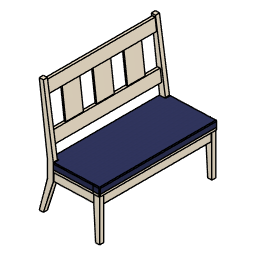
Slatback Bench 2020 (Autodesk Fusion 360 design; units mm, degrees)
Autodesk Fusion 360 part; units mm, degrees
note: some values were not read from the file. Chosen so that the rebuilt part matches the saved one: a direction. Set by a fixed rule: which sketch regions a step uses.
sketch "Sketch1" plane through (0, 0, 0) normal (0, 0, 1) x (1, 0, 0) in component "RearPost"
  line L0 (0, 0) -> (34.925, 0)
  line L1 (121.1545, 271.4692) -> (121.1545, 417.6082)
  line L2 (34.925, 990.6) -> (0, 990.6)
  line L3 (0, 990.6) -> (0, 0)
  line L4 (34.925, 990.6) -> (121.1545, 417.6082)
  line L5 (121.1545, 271.4692) -> (34.925, 0)
  line L6 (34.925, 990.6) -> (34.925, 0) construction
  line L7 (108.7337, 990.6) -> (34.925, 990.6) construction
  line L8 (34.925, 0) -> (111.2989, 0) construction
  line L9 (121.1545, 417.6082) -> (108.7337, 990.6) construction
  line L10 (111.2989, 0) -> (121.1545, 271.4692) construction
  line L11 (0, 990.6) -> (70.3545, 417.6082)
  line L12 (70.3545, 417.6082) -> (70.3545, 271.4692)
  line L13 (70.3545, 271.4692) -> (0, 0)
  line L14 (121.1545, 271.4692) -> (70.3545, 271.4692) construction
  line L15 (70.3545, 417.6082) -> (121.1545, 417.6082) construction
  dimension "d89" = 990.6
  dimension "d91" = 34.925
  dimension "d95" = 417.6082
  dimension "d97" = 50.8
  dimension "d189" = 121.1545
  dimension "d266" = 0
  dimension "d267" = 0
  dimension "d268" = 0
  dimension "d269" = 0
  dimension "d500" = 0
  dimension "d501" = 0
  dimension "d502" = 0
  dimension "d503" = 0
  dimension "d512" = 0
  dimension "d513" = 0
  dimension "d514" = 0
  dimension "d515" = 0
  dimension "d554" = 0
  dimension "d555" = 0
  dimension "d556" = 0
  dimension "d557" = 0
  dimension "d908" = 7
  constraint horizontal L0
  constraint horizontal L2
  constraint vertical L3
  constraint coincident L0.start L3.end
  constraint perpendicular L0 L6
  constraint horizontal L7
  constraint horizontal L8
  constraint perpendicular L2 L12
  constraint horizontal L15
  constraint horizontal L14
  measures "d89" distance of L0.start L2.end
  measures "d91" distance of L2.end L2.start
  measures "d95" distance of L0 L1.end
  measures "d97" distance of L1 L12
  measures "d189" distance of L1 L3
  measures "d908" angle of L3 L11
extrude "Extrude1" add sketch "Sketch1" along normal blind 34.925 contours L0 L1 L2 L4 L5 L11 L12 L13 makes body 1 in component "RearPost"
ref_plane "WorkPlane1" through (60.5773, 495.3, 17.4625) normal (0, 0, 1) x (1, 0, 0) in component "RearPost"
ref_plane "WorkPlane2" through (121.1545, 419.9193, 17.4625) normal (-0.000175, 0, 1) x (0, 1, 0) in component "RearPost"
sketch "Sketch1 (1)" plane through (121.1545, 419.9193, 17.4625) normal (-0.000175, 0, 1) x (0, 1, 0) in component "RearPost"
  line L0 (-606.7514, 0) -> (606.7514, 0)
  line L1 (-142.0963, 0) -> (-142.9054, 23.1684)
  line L2 (-142.9054, 23.1684) -> (-79.444, 25.3845)
  line L3 (-79.444, 25.3845) -> (-78.5576, 0)
  line L4 (-78.5576, 0) -> (-77.6711, -25.3845)
  line L5 (-77.6711, -25.3845) -> (-141.1325, -27.6006)
  line L6 (-141.1325, -27.6006) -> (-142.0963, 0)
  line L7 (-148.4502, 0.003) -> (-148.4502, -0.003)
  dimension "d221" = 92
  dimension "d224" = 63.5
  dimension "d237" = 25.4
  dimension "d574" = 25.4
  constraint coincident L0 L1.start
  constraint perpendicular L1 L2
  constraint coincident L0 L3.end
  constraint perpendicular L2 L3
  constraint perpendicular L4 L5
  constraint parallel L1 L6
  constraint parallel L3 L4
  measures "d221" angle of L0 L1
  measures "d224" distance of L1.end L2.end
  measures "d237" distance of L2.end L3.end
  measures "d574" distance of L3.end L4.end
extrude "Extrude2" cut sketch "Sketch1 (1)" along normal mid plane 12.7 bodies 1 in component "RearPost"
sketch "Sketch3" plane through (0, 0, 0) normal (0, 0, -1) x (-1, 0, 0) in component "RearPost"
  line L0 (0, 990.6) -> (-34.925, 990.6)
  line L1 (-34.925, 990.6) -> (-121.1545, 417.6082)
  line L2 (-121.1545, 417.6082) -> (-121.1545, 271.4692)
  line L3 (-121.1545, 271.4692) -> (-34.925, 0)
  line L4 (-34.925, 0) -> (0, 0)
  line L5 (0, 0) -> (-70.3545, 271.4692)
  line L6 (-70.3545, 271.4692) -> (-70.3545, 417.6082)
  line L7 (-70.3545, 417.6082) -> (0, 990.6)
  line L8 (-121.1545, 271.4692) -> (-70.3545, 271.4692) construction
  line L9 (-94.167, 341.3192) -> (-81.467, 341.3192)
  line L10 (-81.467, 341.3192) -> (-81.467, 277.8192)
  line L11 (-81.467, 277.8192) -> (-94.167, 277.8192)
  line L12 (-94.167, 277.8192) -> (-94.167, 341.3192)
  dimension "d110" = 11.1125
  dimension "d111" = 12.7
  dimension "d112" = 6.35
  dimension "d113" = 63.5
  constraint coincident L2.end L3.start
  constraint coincident L5.end L6.start
  constraint horizontal L9
  constraint vertical L10
  constraint horizontal L11
  constraint vertical L12
  measures "d110" distance of L6 L10
  measures "d111" distance of L9.start L9.end
  measures "d112" distance of L8 L11
  measures "d113" distance of L9.end L10.end
extrude "Extrude3" cut sketch "Sketch3" against normal blind 25.4 contours L9 L10 L11 L12 bodies 1 in component "RearPost"
sketch "Sketch2" plane through (0, 0, 0) normal (0, 0, -1) x (-1, 0, 0) in component "RearPost"
  line L0 (-81.467, 341.3192) -> (-81.467, 277.8192)
  line L1 (-81.467, 277.8192) -> (-94.167, 277.8192)
  line L2 (-94.167, 277.8192) -> (-94.167, 341.3192)
  line L3 (-94.167, 341.3192) -> (-81.467, 341.3192)
  line L4 (0, 990.6) -> (-34.925, 990.6)
  line L5 (-34.925, 990.6) -> (-121.1545, 417.6082)
  line L6 (-121.1545, 417.6082) -> (-121.1545, 271.4692)
  line L7 (-121.1545, 271.4692) -> (-34.925, 0)
  line L8 (-34.925, 0) -> (0, 0)
  line L9 (0, 0) -> (-70.3545, 271.4692)
  line L10 (-70.3545, 271.4692) -> (-70.3545, 417.6082)
  line L11 (-70.3545, 417.6082) -> (0, 990.6)
  line L12 (-81.6076, 521.3529) -> (-70.7734, 609.5902)
  line L13 (-70.7734, 609.5902) -> (-58.1681, 608.0425)
  line L14 (-58.1681, 608.0425) -> (-69.0023, 519.8052)
  line L15 (-69.0023, 519.8052) -> (-81.6076, 521.3529)
  line L16 (-121.1545, 417.6082) -> (-70.3545, 417.6082) construction
  line L17 (-69.0023, 519.8052) -> (-81.3842, 418.9625) construction
  line L18 (-37.5647, 880.054) -> (-26.7305, 968.2913)
  line L19 (-14.1252, 966.7436) -> (-24.9593, 878.5062)
  line L20 (-26.7305, 968.2913) -> (-14.1252, 966.7436)
  line L21 (-24.9593, 878.5062) -> (-37.5647, 880.054)
  line L22 (-58.1681, 608.0425) -> (-24.9593, 878.5062) construction
  line L23 (-14.1252, 966.7436) -> (-11.0297, 991.9543) construction
  line L24 (-70.3545, 417.6082) -> (-81.3842, 418.9625) construction
  line L25 (0, 990.6) -> (-11.0297, 991.9543) construction
  dimension "d852" = 12.7
  dimension "d853" = 88.9
  dimension "d854" = 101.6
  dimension "d857" = 11.1125
  dimension "d860" = 12.7
  dimension "d861" = 88.9
  dimension "d862" = 25.4
  constraint perpendicular L12 L13
  constraint perpendicular L13 L14
  constraint perpendicular L14 L15
  constraint parallel L11 L14
  constraint coincident L5.end L6.start
  constraint coincident L10.end L11.start
  constraint perpendicular L15 L17
  constraint perpendicular L18 L20
  constraint perpendicular L19 L20
  constraint perpendicular L19 L21
  constraint collinear L14 L22
  constraint collinear L19 L22
  constraint perpendicular L20 L23
  constraint perpendicular L11 L24
  constraint coincident L17.end L24.end
  constraint coincident L4.start L11.end
  constraint perpendicular L11 L25
  constraint coincident L23.end L25.end
  measures "d852" distance of L12 L14
  measures "d853" distance of L13.end L14.end
  measures "d854" distance of L14.end L17.end
  measures "d857" distance of L11 L14
  measures "d860" distance of L18 L19
  measures "d861" distance of L19.start L19.end
  measures "d862" distance of L19.start L23.end
extrude "Extrude3'" cut sketch "Sketch2" against normal blind 25.4 contours L12 L13 L14 L15 | L18 L19 L20 L21 bodies 1 in component "RearPost"
sketch "Sketch1 (2)" plane through (0, 0, 0) normal (0, 0, 1) x (1, 0, 0) in component "SideRail"
  line L0 (0, 0) -> (349.4629, 0)
  line L1 (349.4629, 0) -> (352.1238, 76.2)
  line L2 (352.1238, 76.2) -> (2.661, 76.2)
  line L3 (2.661, 76.2) -> (0, 0)
  dimension "d116" = 349.4629
  dimension "d169" = 88
  dimension "d209" = 76.2
  dimension "d262" = 0
  dimension "d263" = 0
  dimension "d264" = 0
  dimension "d265" = 0
  dimension "d496" = 0
  dimension "d497" = 0
  dimension "d498" = 0
  dimension "d499" = 0
  dimension "d508" = 0
  dimension "d509" = 0
  dimension "d510" = 0
  dimension "d511" = 0
  dimension "d550" = 0
  dimension "d551" = 0
  dimension "d552" = 0
  dimension "d553" = 0
  constraint horizontal L0
  constraint horizontal L2
  constraint coincident L0.start L3.end
  constraint parallel L1 L3
  measures "d116" distance of L0.start L0.end
  measures "d169" angle of L0 L3
  measures "d209" distance of L0 L2
sketch "Sketch4" plane through (0, 0, 0) normal (0, 1, 0) x (1, 0, 0) in component "SideRail"
  line L0 (0, 0) -> (-0.0044, 25.4)
  line L1 (352.1238, 0) -> (2.661, 0)
  line L2 (0, 0) -> (0, 25.4) construction
  line L3 (0, 25.4) -> (-0.0044, 25.4) construction
  dimension "d210" = 90.01
  dimension "d217" = 25.4
  constraint coincident L0.start L2.start
  constraint vertical L2
  constraint horizontal L3
  measures "d210" angle of L0 L1
  measures "d217" distance of L0.start L2.end
sweep "Sweep1" add profiles "Sketch1 (2)" path "Sketch4" along L0 section 1 separate body makes body 2 in component "SideRail"
ref_plane "WorkPlane2" through (176.0575, 38.1, -12.7) normal (0, 0, -1) x (-1, 0, 0) in component "SideRail"
sketch "Sketch3 (2)" plane through (179.1297, 38.0768, -12.7) normal (0, 0, -1) x (1, 0, 0) in component "SideRail"
  line L0 (-178.9101, 31.7268) -> (-202.0927, 31.7268)
  line L1 (-202.0927, 31.7268) -> (-202.0927, -31.7732)
  line L2 (-202.0927, -31.7732) -> (-176.6927, -31.7732)
  line L3 (170.5527, 31.7268) -> (195.9527, 31.7268)
  line L4 (195.9527, 31.7268) -> (195.9527, -31.7732)
  line L5 (195.9527, -31.7732) -> (172.7702, -31.7732)
  line L6 (172.9942, -38.1232) -> (172.9897, -38.1232)
  line L7 (170.3332, 38.0768) -> (170.3288, 38.0768)
  line L8 (172.992, -38.1232) -> (170.331, 38.0768)
  line L9 (-176.4687, -38.1232) -> (-176.4731, -38.1232)
  line L10 (-179.1297, 38.0768) -> (-179.1341, 38.0768)
  line L11 (-176.4709, -38.1232) -> (-179.1319, 38.0768)
  line L12 (-176.6927, -31.7732) -> (172.7702, -31.7732)
  line L13 (170.5527, 31.7268) -> (-178.9101, 31.7268)
  line L14 (195.9527, -31.7732) -> (195.9527, -38.1232)
  line L15 (195.9527, -38.1232) -> (160.4613, -38.1232)
  line L16 (160.4613, -38.1232) -> (160.4613, -31.7732)
  dimension "d274" = 25.4
  dimension "d325" = 6.35
  dimension "d326" = 6.35
  constraint perpendicular L0 L1
  constraint perpendicular L1 L2
  constraint perpendicular L3 L4
  constraint perpendicular L4 L5
  constraint collinear L0 L3
  constraint collinear L2 L5
  constraint equal L0 L5
  constraint horizontal L2
  constraint midpoint L6 L8.start
  constraint midpoint L7 L8.end
  constraint coincident L3.start L8
  constraint coincident L5.end L8
  constraint midpoint L9 L11.start
  constraint midpoint L10 L11.end
  constraint coincident L2.end L11
  constraint coincident L0.start L11
  constraint perpendicular L5 L14
  constraint perpendicular L14 L15
  constraint coincident L12 L16.end
  constraint perpendicular L12 L16
  constraint coincident L8.start L15
  measures "d274" distance of L1.end L2.end
  measures "d325" distance of L0 L11.end
  measures "d326" distance of L2 L11.start
extrude "Extrude3''" add sketch "Sketch3 (2)" along normal mid plane 12.7 bodies 2 in component "SideRail"
sketch "Sketch4 (2)" plane through (0, 0, 0) normal (0, 0, 1) x (1, 0, 0) in component "FrontPost"
  line L0 (0, 0) -> (34.925, 0)
  line L1 (50.8, 0) -> (50.8, 283.9296) construction
  line L2 (50.8, 360.176) -> (0, 361.95)
  line L3 (0, 361.95) -> (0, 0)
  line L4 (50.8, 283.9296) -> (34.925, 0)
  line L5 (50.8, 283.9296) -> (50.8, 360.176)
  line L6 (34.925, 0) -> (50.8, 0) construction
  dimension "d137" = 361.95
  dimension "d139" = 34.925
  dimension "d140" = 76.2464
  dimension "d190" = 88
  dimension "d191" = 50.8
  dimension "d316" = 50.831
  constraint horizontal L0
  constraint vertical L1
  constraint vertical L3
  constraint coincident L0.start L3.end
  constraint vertical L5
  constraint horizontal L6
  measures "d137" distance of L0.start L2.end
  measures "d139" distance of L0.start L0.end
  measures "d140" distance of L2.start L1.end
  measures "d190" angle of L2 L3
  measures "d191" distance of L3 L5
  measures "d316" distance of L2.start L2.end
extrude "Extrude1'" add sketch "Sketch4 (2)" along normal blind 34.925 separate body makes body 3 in component "FrontPost"
ref_plane "WorkPlane1" through (25.4, 180.975, 17.4625) normal (0, 0, 1) x (1, 0, 0) in component "FrontPost"
ref_plane "WorkPlane2" through (50.8, 251.5139, 17.4625) normal (-0.000175, 0, 1) x (0, 1, 0) in component "FrontPost"
sketch "Sketch2 (2)" plane through (50.8, 251.5139, 17.4625) normal (-0.000175, 0, 1) x (0, 1, 0) in component "FrontPost"
  line L0 (94.9658, 0) -> (95.7838, 23.4252)
  line L1 (95.7838, 23.4252) -> (39.6773, 25.3845)
  line L2 (39.6773, 25.3845) -> (38.7908, 0)
  line L3 (-204.4066, 0) -> (204.4066, 0)
  line L4 (94.9658, 0) -> (94.7884, -5.08)
  line L5 (94.7884, -5.08) -> (38.6134, -5.08)
  line L6 (38.6134, -5.08) -> (38.7908, 0)
  line L7 (146.522, 21.6534) -> (145.5884, -5.08)
  line L8 (94.7884, -5.08) -> (145.5884, -5.08)
  line L9 (95.7838, 23.4252) -> (146.522, 21.6534)
  line L10 (32.4157, 0.003) -> (32.4157, -0.003)
  dimension "d192" = 25.4
  dimension "d279" = 92
  dimension "d647" = 50.8
  constraint parallel L0 L2
  constraint perpendicular L0 L1
  constraint coincident L2.end L3
  constraint coincident L0.start L3
  constraint parallel L2 L6
  constraint parallel L0 L4
  constraint parallel L5 L8
  constraint horizontal L5
  constraint parallel L1 L9
  constraint parallel L0 L7
  measures "d192" distance of L1.end L2.end
  measures "d279" angle of L0 L3
  measures "d647" distance of L4.end L7.end
extrude "Extrude3'''" cut sketch "Sketch2 (2)" along normal mid plane 12.7 bodies 3 in component "FrontPost"
sketch "Sketch3 (3)" plane through (0, 0, 34.925) normal (0, 0, 1) x (1, 0, 0) in component "FrontPost"
  line L0 (50.8, 283.9296) -> (50.8, 360.176)
  line L1 (50.8, 360.176) -> (0, 361.95)
  line L2 (0, 361.95) -> (0, 0)
  line L3 (0, 0) -> (34.925, 0)
  line L4 (34.925, 0) -> (50.8, 283.9296)
  line L5 (0, 361.95) -> (54.2925, 361.95)
  line L6 (11.1125, 355.6) -> (23.8125, 355.6)
  line L7 (23.8125, 355.6) -> (23.8125, 292.1)
  line L8 (23.8125, 292.1) -> (11.1125, 292.1)
  line L9 (11.1125, 292.1) -> (11.1125, 355.6)
  line L10 (11.1125, 355.6) -> (11.1125, 361.95)
  line L11 (23.8125, 355.6) -> (23.8125, 361.95)
  dimension "d544" = 12.7
  dimension "d545" = 6.35
  dimension "d546" = 63.5
  dimension "d547" = 11.1125
  constraint coincident L1.end L2.start
  constraint perpendicular L2 L5
  constraint horizontal L6
  constraint vertical L7
  constraint horizontal L8
  constraint vertical L9
  constraint coincident L5 L10.end
  constraint perpendicular L5 L10
  constraint coincident L5 L11.end
  constraint perpendicular L5 L11
  measures "d544" distance of L6.start L6.end
  measures "d545" distance of L5 L6
  measures "d546" distance of L6.start L8.end
  measures "d547" distance of L2 L9
extrude "Extrude4" cut sketch "Sketch3 (3)" against normal blind 25.4 contours L1 L6 L10 L11 | L1 L5 L10 L11 | L6 L7 L8 L9 bodies 3 in component "FrontPost"
sketch "Sketch3 (4)" plane through (0, 0, 0) normal (0, 0, 1) x (1, 0, 0) in component "FrontRail"
  line L0 (0, 0) -> (0, 74.925)
  line L1 (0, 74.925) -> (25.4, 75.8119)
  line L2 (25.4, 75.8119) -> (25.4, 0)
  line L3 (25.4, 0) -> (0, 0)
  line L4 (36.5125, 0) -> (36.5125, 76.2) construction
  line L5 (36.5125, 76.2) -> (-4.1275, 76.2) construction
  dimension "d669" = 25.4
  dimension "d670" = 11.1125
  dimension "d671" = 88
  dimension "d672" = 76.2
  constraint coincident L0.start L3.end
  constraint vertical L0
  constraint parallel L0 L2
  constraint perpendicular L0 L3
  constraint vertical L4
  constraint perpendicular L4 L5
  constraint coincident L1 L4.end
  constraint coincident L3 L4.start
  measures "d669" distance of L2.end L0.start
  measures "d670" distance of L2 L4
  measures "d671" angle of L1 L2
  measures "d672" distance of L4.start L4.end
extrude "Extrude3''''" add sketch "Sketch3 (4)" along normal blind 933.45 separate body makes body 4 in component "FrontRail"
ref_plane "WorkPlane2" through (12.7, 37.906, 466.725) normal (0, 0, 1) x (1, 0, 0) in component "FrontRail"
sketch "Sketch4 (3)" plane through (0, 0, 933.45) normal (0, 0, 1) x (1, 0, 0) in component "FrontRail"
  line L0 (25.4, 0) -> (25.4, 75.8119)
  line L1 (25.4, 75.8119) -> (0, 74.925)
  line L2 (0, 74.925) -> (0, 0)
  line L3 (0, 0) -> (25.4, 0)
  line L4 (6.35, 75.1467) -> (6.35, 6.35)
  line L5 (6.35, 6.35) -> (19.05, 6.35)
  line L6 (19.05, 6.35) -> (19.05, 75.5902)
  line L7 (12.7, 75.3685) -> (12.7, 0) construction
  point P0 (12.7, 6.35)
  dimension "d675" = 12.7
  dimension "d676" = 6.35
  constraint coincident L1 L4.start
  constraint parallel L0 L4
  constraint perpendicular L4 L5
  constraint coincident L1 L6.end
  constraint perpendicular L5 L6
  constraint midpoint L1 L7.start
  constraint midpoint L3 L7.end
  constraint midpoint L5 P0
  constraint coincident L7 P0
  measures "d675" distance of L4.end L5.end
  measures "d676" distance of L3 L5
extrude "Extrude4'" add sketch "Sketch4 (3)" along normal blind 25.4 contours L1 L4 L5 L6 bodies 4 in component "FrontRail"
mirror "Mirror2" about plane through (12.7, 37.906, 466.725) normal (0, 0, 1) of "Extrude4'" in component "FrontRail"
sketch "Sketch1 (3)" plane through (0, 0, 0) normal (0, 0, 1) x (1, 0, 0) in component "RearRail"
  line L0 (0, 0) -> (0, 74.8605)
  line L1 (0, 74.8605) -> (25.4, 75.7475)
  line L2 (25.4, 75.7475) -> (25.4, 0)
  line L3 (25.4, 0) -> (0, 0)
  line L4 (-11.1125, 113.0857) -> (-11.1125, 0) construction
  line L5 (-11.1125, 0) -> (39.6875, 0) construction
  line L6 (-11.1125, 113.0857) -> (39.6875, 113.0857) construction
  line L7 (39.6875, 0) -> (39.6875, 76.2464) construction
  line L8 (39.6875, 76.2464) -> (39.6875, 113.0857) construction
  dimension "d752" = 25.4
  dimension "d753" = 88
  dimension "d755" = 11.1125
  dimension "d756" = 50.8
  dimension "d757" = 76.2464
  constraint coincident L0.start L3.end
  constraint vertical L0
  constraint parallel L0 L2
  constraint perpendicular L0 L3
  constraint parallel L0 L4
  constraint perpendicular L4 L5
  constraint perpendicular L4 L6
  constraint collinear L3 L5
  constraint perpendicular L6 L8
  constraint coincident L1 L7.end
  constraint collinear L7 L8
  measures "d752" distance of L2.end L0.start
  measures "d753" angle of L1 L2
  measures "d755" distance of L0 L4
  measures "d756" distance of L4.end L5.end
  measures "d757" distance of L5.end L7.end
extrude "Extrude1''" add sketch "Sketch1 (3)" along normal blind 933.328 separate body makes body 5 in component "RearRail"
ref_plane "WorkPlane1" through (12.7, 37.8738, 466.664) normal (0, 0, 1) x (1, 0, 0) in component "RearRail"
sketch "Sketch2 (3)" plane through (0, 0, 933.328) normal (0, 0, 1) x (1, 0, 0) in component "RearRail"
  line L0 (25.4, 0) -> (25.4, 75.7475)
  line L1 (25.4, 75.7475) -> (0, 74.8605)
  line L2 (0, 74.8605) -> (0, 0)
  line L3 (0, 0) -> (25.4, 0)
  line L4 (6.35, 6.35) -> (19.05, 6.35)
  line L5 (19.05, 6.35) -> (19.05, 69.85)
  line L6 (19.05, 69.85) -> (6.35, 69.85)
  line L7 (6.35, 69.85) -> (6.35, 6.35)
  line L8 (12.7, 0) -> (12.7, 75.304) construction
  point P0 (12.7, 6.35)
  dimension "d760" = 6.35
  dimension "d761" = 12.7
  dimension "d762" = 63.5
  constraint horizontal L4
  constraint vertical L5
  constraint horizontal L6
  constraint vertical L7
  constraint midpoint L3 L8.start
  constraint midpoint L1 L8.end
  constraint midpoint L4 P0
  constraint coincident L8 P0
  measures "d760" distance of L3 L4
  measures "d761" distance of L4.start L4.end
  measures "d762" distance of L4.end L5.end
extrude "Extrude2'" add sketch "Sketch2 (3)" along normal blind 25.4 contours L4 L5 L6 L7 bodies 5 in component "RearRail"
mirror "Mirror1" about plane through (12.7, 37.8738, 466.664) normal (0, 0, 1) of "Extrude2'" in component "RearRail"
sketch "Sketch1 (4)" plane through (0, 0, 0) normal (0, 1, 0) x (1, 0, 0) in component "Seat"
  line L0 (0, 0) -> (52.4194, 0)
  line L1 (52.4194, 0) -> (52.4194, -41.275)
  line L2 (52.4194, -41.275) -> (401.9172, -41.336)
  line L3 (401.9172, 974.664) -> (52.4194, 974.603)
  line L4 (52.4194, 974.603) -> (52.4194, 933.328)
  line L5 (52.4194, 933.328) -> (0, 933.328)
  line L6 (0, 933.328) -> (0, 0)
  line L7 (401.9172, -41.336) -> (459.0672, -41.336)
  line L8 (459.0672, -41.336) -> (459.0672, 974.664)
  line L9 (459.0672, 974.664) -> (401.9172, 974.664)
  line L10 (401.9172, -41.336) -> (401.9172, 974.664) construction
  dimension "d780" = 90.01
  dimension "d781" = 90.01
  dimension "d785" = 933.328
  dimension "d786" = 52.4194
  dimension "d787" = 57.15
  dimension "d789" = 406.6477
  dimension "d790" = 1016
  constraint coincident L0.start L6.end
  constraint horizontal L0
  constraint perpendicular L0 L1
  constraint perpendicular L0 L6
  constraint collinear L1 L4
  constraint perpendicular L5 L6
  constraint equal L1 L4
  constraint perpendicular L7 L8
  constraint perpendicular L8 L9
  constraint parallel L8 L10
  constraint parallel L6 L8
  measures "d780" angle of L1 L2
  measures "d781" angle of L3 L4
  measures "d785" distance of L5.end L0.start
  measures "d786" distance of L0.start L0.end
  measures "d787" horizontal distance of L2.end L7.end
  measures "d789" distance of L1 L8
  measures "d790" distance of L7.end L8.end
sketch "Sketch2 (4)" plane through (0, 0, 0) normal (0, 0, 1) x (1, 0, 0) in component "Seat"
  line L0 (0, 0) -> (0.6652, 19.05)
  line L1 (0, 0) -> (0.045, 1.2883)
  line L2 (0, 19.05) -> (0.6652, 19.05) construction
  line L3 (0, 19.05) -> (0, 0) construction
  dimension "d791" = 19.05
  dimension "d792" = 2
  constraint coincident L0.start L1.start
  constraint coincident L0 L1.end
  constraint vertical L3
  constraint perpendicular L2 L3
  measures "d791" distance of L2.start L0.start
  measures "d792" angle of L0 L3
sweep "Sweep1'" add profiles "Sketch1 (4)" path "Sketch2 (4)" along L0 section 1 separate body makes body 6 in component "Seat"
fillet "Fillet1" radius 6.35 6 edges at (459.3998, 9.525, 41.336) (52.7521, 9.525, 41.275) (459.3998, 9.525, -974.664) (52.7521, 9.525, -974.603) (0.3326, 9.525, -933.328) (0.3326, 9.525, 0) on bodies 6 in component "Seat"
sketch "Sketch1 (5)" plane through (0, 0, 0) normal (0, 1, 0) x (1, 0, 0) in component "Cushion"
  line L0 (0, 0) -> (52.4194, 0)
  line L1 (52.4194, 0) -> (52.4194, -41.275)
  line L2 (52.4194, -41.275) -> (401.9172, -41.336)
  line L3 (401.9172, 974.664) -> (52.4194, 974.603)
  line L4 (52.4194, 974.603) -> (52.4194, 933.328)
  line L5 (52.4194, 933.328) -> (0, 933.328)
  line L6 (0, 933.328) -> (0, 0)
  line L7 (401.9172, -41.336) -> (459.0672, -41.336)
  line L8 (459.0672, -41.336) -> (459.0672, 974.664)
  line L9 (459.0672, 974.664) -> (401.9172, 974.664)
  line L10 (401.9172, -41.336) -> (401.9172, 974.664) construction
  dimension "d780_1" = 90.01
  dimension "d781_1" = 90.01
  dimension "d785_1" = 933.328
  dimension "d786_1" = 52.4194
  dimension "d787_1" = 57.15
  dimension "d789_1" = 406.6477
  dimension "d790_1" = 1016
  constraint coincident L0.start L6.end
  constraint horizontal L0
  constraint perpendicular L0 L1
  constraint perpendicular L0 L6
  constraint collinear L1 L4
  constraint perpendicular L5 L6
  constraint equal L1 L4
  constraint perpendicular L7 L8
  constraint perpendicular L8 L9
  constraint parallel L8 L10
  constraint parallel L6 L8
  measures "d780_1" angle of L1 L2
  measures "d781_1" angle of L3 L4
  measures "d785_1" distance of L5.end L0.start
  measures "d786_1" distance of L0.start L0.end
  measures "d787_1" horizontal distance of L2.end L7.end
  measures "d789_1" distance of L1 L8
  measures "d790_1" distance of L7.end L8.end
sketch "Sketch2 (5)" plane through (0, 0, 0) normal (0, 0, 1) x (1, 0, 0) in component "Cushion"
  line L0 (0, 0) -> (1.774, 50.8)
  line L1 (0, 0) -> (0.045, 1.2883)
  line L2 (0, 50.8) -> (1.774, 50.8) construction
  line L3 (0, 50.8) -> (0, 0) construction
  dimension "d791_1" = 50.8
  dimension "d792_1" = 2
  constraint coincident L0.start L1.start
  constraint coincident L0 L1.end
  constraint vertical L3
  constraint perpendicular L2 L3
  measures "d791_1" distance of L2.start L0.start
  measures "d792_1" angle of L0 L3
sweep "Sweep1''" add profiles "Sketch1 (5)" path "Sketch2 (5)" along L0 section 1 separate body makes body 7 in component "Cushion"
fillet "Fillet1'" radius 6.35 16 edges at (228.9423, 50.8, 41.3055) (432.2661, 50.8, 41.336) (460.8411, 50.8, -466.664) (432.2661, 50.8, -974.664) (228.9423, 50.8, -974.6335) (54.1934, 50.8, -953.9655) (27.9837, 50.8, -933.328) (1.774, 50.8, -466.664) (27.9837, 50.8, 0) (54.1934, 50.8, 20.6375) (459.9541, 25.4, -974.664) (53.3064, 25.4, -974.603) (459.9541, 25.4, 41.336) (53.3064, 25.4, 41.275) (0.887, 25.4, 0) (0.887, 25.4, -933.328) on bodies 7 in component "Cushion"
sketch "Sketch1 (6)" plane through (0, 0, 0) normal (0, 1, 0) x (1, 0, 0) in component "BackRail"
  line L0 (0, 0) -> (25.4, 0)
  line L1 (25.4, 0) -> (25.4, -933.328)
  line L2 (25.4, -933.328) -> (0, -933.328)
  line L3 (0, -933.328) -> (0, 0)
  dimension "d940" = 933.328
  dimension "d941" = 25.4
  constraint horizontal L0
  constraint vertical L1
  constraint horizontal L2
  constraint vertical L3
  constraint coincident L0.start L3.end
  measures "d940" distance of L0.end L1.end
  measures "d941" distance of L0.start L0.end
extrude "Extrude1'''" add sketch "Sketch1 (6)" along normal blind 101.6 separate body makes body 8 in component "BackRail"
ref_plane "WorkPlane1" through (12.7, 50.8, 466.664) normal (0, 0, 1) x (1, 0, 0) in component "BackRail"
sketch "Sketch2 (6)" plane through (0, 0, 933.328) normal (0, 0, 1) x (1, 0, 0) in component "BackRail"
  line L0 (6.35, 95.25) -> (19.05, 95.25)
  line L1 (19.05, 95.25) -> (19.05, 6.35)
  line L2 (19.05, 6.35) -> (6.35, 6.35)
  line L3 (6.35, 6.35) -> (6.35, 95.25)
  line L4 (0, 0) -> (25.4, 101.6) construction
  line L5 (6.35, 95.25) -> (19.05, 6.35) construction
  line L6 (0, 101.6) -> (25.4, 101.6)
  point P0 (25.4, 101.6)
  dimension "d871" = 12.7
  dimension "d942" = 6.35
  constraint horizontal L0
  constraint vertical L1
  constraint horizontal L2
  constraint vertical L3
  constraint midpoint L4 L5
  constraint coincident L4.start origin
  constraint coincident P0 L4.end
  measures "d871" distance of L1.end L2.end
  measures "d942" distance of L0 L6
extrude "Extrude2''" add sketch "Sketch2 (6)" along normal blind 25.4 bodies 8 in component "BackRail"
mirror "Mirror1'" about plane through (12.7, 50.8, 466.664) normal (0, 0, 1) of "Extrude2''" in component "BackRail"
sketch "Sketch3 (5)" plane through (0, 101.6, 0) normal (0, 1, 0) x (-1, 0, 0) in component "BackRail"
  line L0 (0, 933.328) -> (-25.4, 933.328)
  line L1 (-25.4, 933.328) -> (-25.4, 0)
  line L2 (-25.4, 0) -> (0, 0)
  line L3 (0, 0) -> (0, 933.328)
  line L4 (-9.525, 539.689) -> (-15.875, 539.689)
  line L5 (-15.875, 539.689) -> (-15.875, 393.639)
  line L6 (-15.875, 393.639) -> (-9.525, 393.639)
  line L7 (-9.525, 393.639) -> (-9.525, 539.689)
  line L8 (-12.7, 933.328) -> (-12.7, 0) construction
  line L9 (-9.525, 539.689) -> (-15.875, 393.639) construction
  line L10 (-15.875, 660.339) -> (-9.525, 660.339)
  line L11 (-9.525, 806.389) -> (-15.875, 806.389)
  line L12 (-15.875, 806.389) -> (-15.875, 660.339)
  line L13 (-9.525, 806.389) -> (-15.875, 660.339) construction
  line L14 (-9.525, 660.339) -> (-9.525, 806.389)
  line L15 (-15.875, 126.939) -> (-9.525, 126.939)
  line L16 (-9.525, 272.989) -> (-15.875, 272.989)
  line L17 (-15.875, 272.989) -> (-15.875, 126.939)
  line L18 (-9.525, 272.989) -> (-15.875, 126.939) construction
  line L19 (-9.525, 126.939) -> (-9.525, 272.989)
  point P0 (-25412.7042, 466.725)
  point P1 (-25412.7042, 466.664)
  dimension "d943" = 6.35
  dimension "d944" = 146.05
  dimension "d947" = 266.7
  dimension "d948" = 0
  constraint horizontal L4
  constraint vertical L5
  constraint horizontal L6
  constraint vertical L7
  constraint midpoint L0 L8.start
  constraint midpoint L2 L8.end
  constraint midpoint L8 L9
  measures "d943" distance of L4.start L4.end
  measures "d944" distance of L4.start L6.end
extrude "Extrude3'''''" cut sketch "Sketch3 (5)" against normal blind 12.7 contours L4 L5 L6 L7 | L10 L11 L12 L14 | L15 L16 L17 L19 bodies 8 in component "BackRail"
sketch "Sketch1 (7)" plane through (0, 0, 0) normal (0, 1, 0) x (1, 0, 0) in component "BackPanel"
  line L0 (0.0114, 0) -> (12.7114, 0)
  line L1 (12.7114, 0) -> (12.7114, -152.4) construction
  line L2 (12.7114, -152.4) -> (0.0114, -152.4)
  line L3 (0, -152.4) -> (0, 0) construction
  arc A0 (12.7114, 0) -> (12.7114, -152.4) centre (254006.35, -76.2) ccw
  arc A1 (0.0114, 0) -> (0.0114, -152.4) centre (254006.35, -76.2) ccw
  line L4 (0, 0) -> (0.0114, 0) construction
  line L5 (0.0114, -152.4) -> (0, -152.4) construction
  arc A2 (6.3614, 0) -> (6.3614, -152.4) centre (254006.35, -76.2) ccw construction
  dimension "d910" = 152.4
  dimension "d911" = 254000
  dimension "d912" = 12.7
  constraint horizontal L0
  constraint vertical L1
  constraint horizontal L2
  constraint vertical L3
  constraint coincident L3.end L4.start
  constraint tangent L3 A1
  constraint concentric A0 A1
  constraint horizontal L4
  constraint horizontal L5
  constraint midpoint L2 A2.end
  constraint midpoint L0 A2.start
  constraint concentric A1 A2
  measures "d910" distance of L0.end L1.end
  measures "d911" radius of A2
  measures "d912" distance of L1.end L2.end
extrude "Extrude1''''" add sketch "Sketch1 (7)" along normal blind 259.7949 separate body makes body 9 in component "BackPanel"
ref_plane "WorkPlane1" through (6.35, 129.8974, 76.2) normal (0, 1, 0) x (1, 0, 0) in component "BackPanel"
sketch "Sketch2 (7)" plane through (0, 259.7949, 0) normal (0, 1, 0) x (-1, 0, 0) in component "BackPanel"
  line L0 (-12.7114, 0) -> (-0.0114, 0)
  arc A0 (-0.0114, 0) -> (-0.0114, 152.4) centre (-254006.35, 76.2) ccw
  line L1 (-0.0114, 152.4) -> (-12.7114, 152.4)
  arc A1 (-12.7114, 0) -> (-12.7114, 152.4) centre (-254006.35, 76.2) ccw
  arc A2 (-9.5355, 3.175) -> (-9.5355, 149.225) centre (-254006.35, 76.2) ccw
  arc A3 (-3.1855, 3.175) -> (-3.1855, 149.225) centre (-254006.35, 76.2) ccw
  line L2 (-3.1855, 149.225) -> (-9.5355, 149.225)
  line L3 (-3.1855, 3.175) -> (-9.5355, 3.175)
  point P0 (-2540006.5048, 76.2)
  point P1 (-25406.35, 76.2)
  point P2 (-254006.3512, 76.2)
  dimension "d917" = 3.175
  dimension "d918" = 3.175
  dimension "d920" = 3.175
  dimension "d936" = 3.175
  constraint horizontal L2
  constraint parallel L2 L3
  constraint concentric A2 A3
  constraint concentric A1 A2
  measures "d917" distance of L1 L2
  measures "d918" distance of L0 L3
  measures "d920" distance of A0 A3
  measures "d936" distance of A1 A2
extrude "Extrude2'''" add sketch "Sketch2 (7)" along normal blind 12.7 contours A2 A3 L2 L3 bodies 9 in component "BackPanel"
mirror "Mirror1''" about plane through (6.35, 129.8974, 76.2) normal (0, 1, 0) of "Extrude2'''" in component "BackPanel"
mirror "MirrorComponent2" about plane through (0, 0, 0) normal (0, 0, 1) of bodies 2 makes body 10 in component "SideRail(Mirror)"
mirror "MirrorComponent2'" about plane through (0, 0, 0) normal (0, 0, 1) of bodies 1 makes body 11 in component "RearPost(Mirror)"
mirror "MirrorComponent2''" about plane through (0, 0, 0) normal (0, 0, 1) of bodies 3 makes body 12 in component "FrontPost(Mirror)"
component "RearPost" placed x (1, 0, 0) y (0, 1, 0) z (0, 0, 1) at (0, 0, 0)
component "SideRail" placed x (0.999391, 0.034899, 0.000174) y (-0.034899, 0.999391, -0.000006) z (-0.000175, 0, 1) at (121.1545, 271.4693, 30.1625)
component "FrontPost" placed x (-1, 0, 0) y (0, 1, 0) z (0, 0, -1) at (521.2045, -0.2856, 34.986)
component "FrontRail" placed x (1, 0, 0) y (0, 1, 0) z (0, 0, 1) at (491.042, 285.5753, -933.389)
component "RearRail" placed x (1, 0, 0) y (0, 1, 0) z (0, 0, 1) at (75.117, 271.4692, -933.328)
component "Seat" placed x (0.999391, 0.034899, 0) y (-0.034899, 0.999391, 0) z (0, 0, 1) at (68.767, 346.108, 0)
component "Cushion" placed x (0.999391, 0.034899, 0) y (-0.034899, 0.999391, 0) z (0, 0, 1) at (68.767, 365.1696, 0)
component "BackRail" placed x (0.992546, 0.121869, 0) y (-0.121869, 0.992546, 0) z (0, 0, 1) at (63.4735, 512.7286, -933.328)
component "BackRail" placed x (0.992546, 0.121869, 0) y (0.121869, -0.992546, 0) z (0, 0, -1) at (7.0486, 972.2724, 0)
component "BackPanel" placed x (0.992546, 0.121869, 0) y (-0.121869, 0.992546, 0) z (0, 0, 1) at (57.3942, 614.3452, -542.864)
component "RearPost(Mirror)" placed x (1, 0, 0) y (0, 1, 0) z (0, 0, 1) at (0, 0, -933.3281)
component "SideRail(Mirror)" placed x (0.999391, 0.034899, -0.000174) y (-0.034899, 0.999391, 0.000006) z (0.000175, 0, 1) at (121.1545, 271.4693, -963.4906)
component "FrontPost(Mirror)" placed x (-1, 0, 0) y (0, 1, 0) z (0, 0, -1) at (521.2045, -0.2856, -968.314)
component "BackPanel" placed x (0.992546, 0.121869, 0) y (-0.121869, 0.992546, 0) z (0, 0, 1) at (57.3942, 614.3452, -276.164)
component "BackPanel" placed x (0.992546, 0.121869, 0) y (-0.121869, 0.992546, 0) z (0, 0, 1) at (57.3942, 614.3452, -809.564)
equation "seat_height = 17 in"
equation "seat_depth = 16 in"
equation "seat_width = 40 in"
equation "back_height = 22 in"
equation "back_angle = 7 deg"
equation "post_thickness = 1.375 in"
equation "rail_width = 3 in"
equation "panel_width = 4 in"
equation "height = seat_height + back_height"
equation "cushion_thickness = 2 in"
equation "seat_thickness = 0.75 in"
equation "shoulder_wideWidth = ( 7 / 16 ) * 1 in"
equation "tenon_length = 1 in"
equation "foot_height = 2 in"
equation "shoulder_narrowWidth = 0.25 in"
equation "seat_taper = 0.01 deg"
equation "d89 = height"
equation "d91 = post_thickness"
equation "d92 = ( rail_width + seat_thickness + cushion_thickness ) / cos(seat_slope)"
equation "d95 = seat_rearHeight"
equation "d97 = post_width"
equation "post_width = 2 in"
equation "d99 = post_thickness"
equation "d102 = shoulder_wideWidth"
equation "tenon_thickness = 0.5 in"
equation "rail_thickness = 1 in"
equation "d110 = shoulder_wideWidth"
equation "d111 = tenon_thickness"
equation "d112 = shoulder_narrowWidth"
equation "d113 = rail_width - 2 * shoulder_narrowWidth"
equation "d116 = sideRail_length"
equation "d137 = seat_height - seat_thickness - cushion_thickness"
equation "d139 = post_thickness"
equation "d140 = rail_width / cos(seat_slope)"
equation "d143 = post_thickness"
equation "seat_slope = 2 deg"
equation "d166 = tenon_thickness"
equation "d169 = 90 deg - seat_slope"
equation "d175 = tenon_thickness"
equation "d190 = 90 deg - seat_slope"
equation "d191 = post_width"
equation "d192 = tenon_length"
equation "d193 = shoulder_narrowWidth / cos(seat_slope)"
equation "d195 = tenon_thickness"
equation "d209 = rail_width"
equation "d210 = 90 deg + seat_taper"
equation "d217 = rail_thickness"
equation "d220 = -seat_taper"
equation "d221 = 90 deg + seat_slope"
equation "d224 = rail_width - 2 * shoulder_narrowWidth"
equation "d237 = tenon_length"
equation "d274 = tenon_length"
equation "d275 = -seat_taper"
equation "d277 = shoulder_narrowWidth"
equation "d279 = 90 deg + seat_slope"
equation "d325 = shoulder_narrowWidth"
equation "d326 = shoulder_narrowWidth"
equation "d351 = -tenon_length"
equation "d544 = tenon_thickness"
equation "d545 = shoulder_narrowWidth"
equation "d546 = rail_width - 2 * shoulder_narrowWidth"
equation "d547 = shoulder_wideWidth"
equation "d548 = -tenon_length"
equation "d669 = rail_thickness"
equation "d670 = shoulder_wideWidth"
equation "d671 = 90 deg - seat_slope"
equation "d672 = rail_width"
equation "d673 = seat_width - 2 * post_thickness - 2 * seat_overhang"
equation "d675 = tenon_thickness"
equation "d676 = shoulder_narrowWidth"
equation "d677 = tenon_length"
equation "d752 = rail_thickness"
equation "d753 = 90 deg - seat_slope"
equation "d755 = shoulder_wideWidth"
equation "d756 = post_width"
equation "d757 = rail_width / cos(seat_slope)"
equation "d758 = rearRail_length"
equation "d760 = shoulder_narrowWidth"
equation "d761 = tenon_thickness"
equation "d762 = rail_width - 2 * shoulder_narrowWidth"
equation "d763 = tenon_length"
equation "sideRail_length = ( seat_depth - post_width - seat_overhang ) / cos(seat_slope) / cos(seat_taper)"
equation "seat_overhang = 0.25 in"
equation "d780 = 90 deg + seat_taper"
equation "d781 = d780"
equation "d785 = rearRail_length"
equation "d786 = ( post_width - shoulder_wideWidth + seat_overhang + ( rail_thickness - tenon_thickness ) / 2 ) / cos(seat_slope)"
equation "d787 = post_width + seat_overhang"
equation "d789 = seat_depth / cos(seat_slope)"
equation "d790 = seat_width"
equation "d791 = seat_thickness"
equation "d792 = seat_slope"
equation "d780_1 = 90 deg + seat_taper"
equation "d781_1 = d780_1"
equation "d785_1 = rearRail_length"
equation "d786_1 = ( post_width - shoulder_wideWidth + seat_overhang + ( rail_thickness - tenon_thickness ) / 2 ) / cos(seat_slope)"
equation "d787_1 = post_width + seat_overhang"
equation "d789_1 = seat_depth / cos(seat_slope)"
equation "d790_1 = seat_width"
equation "d791_1 = cushion_thickness"
equation "d792_1 = seat_slope"
equation "rearRail_length = seat_width - 2 * post_thickness - 2 * sideRail_length * sin(seat_taper) - 2 * seat_overhang"
equation "d848 = cushion_fillet"
equation "d849 = cushion_fillet"
equation "cushion_fillet = 0.25 in"
equation "d852 = tenon_thickness"
equation "d853 = backRail_width - 2 * shoulder_narrowWidth"
equation "d854 = lumbar_height"
equation "backRail_width = 4 in"
equation "lumbar_height = 4 in"
equation "d857 = shoulder_wideWidth"
equation "d858 = -tenon_length"
equation "d860 = tenon_thickness"
equation "d861 = backRail_width - 2 * shoulder_narrowWidth"
equation "d862 = topRail_offset"
equation "topRail_offset = 1 in"
equation "back_radius = 10000 in"
equation "d869 = backRail_width"
equation "d871 = tenon_thickness"
equation "d873 = tenon_length"
equation "backPanel_width = 6 in"
equation "backPanel_thickness = 0.5 in"
equation "backPanel_shoulder = 0.125 in"
equation "d882 = -backPanel_thickness"
equation "d908 = back_angle"
equation "d910 = backPanel_width"
equation "d911 = back_radius"
equation "d912 = backPanel_thickness"
equation "seat_rearHeight = seat_height - seat_depth * tan(seat_slope)"
equation "backPanel_height = ( height - seat_rearHeight ) / cos(back_angle) - topRail_offset - lumbar_height - 2 * backRail_width + 2 * shoulder_narrowWidth"
equation "d915 = backPanel_height"
equation "d917 = backPanel_shoulder"
equation "d918 = backPanel_shoulder"
equation "d920 = backPanel_shoulder"
equation "d921 = backPanel_thickness"
equation "d936 = backPanel_shoulder"
equation "d940 = rearRail_length"
equation "d941 = rail_thickness"
equation "d942 = shoulder_narrowWidth"
equation "d943 = backPanel_thickness - 2 * backPanel_shoulder"
equation "d944 = backPanel_width - 2 * backPanel_shoulder"
